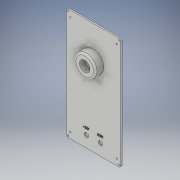
# Autodesk Inventor part: InnerDoorCover
Saved by Autodesk Inventor 2019 (Build 230136000, 136)
## iProperties
Created: 2019-02-25
Part Number: InnerDoorCover
Material: Generic
Document SubType Name: Modeling
Designer: garretthagen21
Density: 1 g/cm^3
Appearance: Default
Author: garretthagen21
Autodesk Inventor part; units mm, degrees
ref_plane "YZ Plane" through (0, 0, 0) normal (1, 0, 0) x (0, 1, 0)
ref_plane "XZ Plane" through (0, 0, 0) normal (0, 1, 0) x (-1, 0, 0)
ref_plane "XY Plane" through (0, 0, 0) normal (0, 0, 1) x (1, 0, 0)
sketch "Base" plane through (0, 0, 0) normal (0, 0, 1) x (1, 0, 0)
  line L0 (-5.5432, 7.38) -> (85.3888, 7.38)
  line L1 (88.5638, 4.205) -> (88.5638, -189.343)
  line L2 (85.3888, -192.518) -> (-5.5432, -192.518)
  line L3 (-8.7182, -189.343) -> (-8.7182, 4.205)
  arc A0 (-5.5432, 7.38) -> (-8.7182, 4.205) centre (-5.5432, 4.205) ccw
  arc A1 (88.5638, 4.205) -> (85.3888, 7.38) centre (85.3888, 4.205) ccw
  arc A2 (85.3888, -192.518) -> (88.5638, -189.343) centre (85.3888, -189.343) ccw
  arc A3 (-8.7182, -189.343) -> (-5.5432, -192.518) centre (-5.5432, -189.343) ccw
  point P0 (0, 0)
  point P1 (88.5638, -192.518)
  point P2 (88.5638, 7.38)
  point P3 (-8.7182, -192.518)
  dimension "d0" = 97.282
  dimension "d1" = 199.898
  dimension "d2" = 3.175
  constraints: 8 end point, 8 point on circle, 8 tangent, 6 point on line, 4 centre point, 3 equal radius, 2 parallel, 1 horizontal, 1 perpendicular
  measures "d0" distance of point (88.564, -192.518) point (-8.718, -192.518)
  measures "d1" distance of point (88.564, 7.38) point (88.564, -192.518)
  measures "d2" radius of A0
extrude "Extrusion1" add sketch "Base" along normal blind 2.54
sketch "Sketch2" plane through (0, 0, 2.54) normal (0, 0, 1) x (1, 0, 0)
  line L0 (85.3888, 7.38) -> (-5.5432, 7.38) projected
  line L1 (-8.7182, 4.205) -> (-8.7182, -189.343) projected
  line L2 (88.5638, -189.343) -> (88.5638, 4.205) projected
  line L3 (-5.5432, -192.518) -> (85.3888, -192.518) projected
  point P0 (0, 0)
  point P1 (-5.4162, 4.078)
  point P2 (85.2618, 4.078)
  point P3 (-5.4162, -189.216)
  point P4 (85.2618, -189.216)
  point P5 (-1.6062, -3.542)
  point P6 (81.4518, -3.542)
  point P7 (81.4518, -181.596)
  point P8 (-1.6062, -181.596)
  dimension "d5" = 3.302
  dimension "d6" = 3.302
  dimension "d7" = 3.302
  dimension "d8" = 3.302
  dimension "d9" = 3.302
  dimension "d10" = 3.302
  dimension "d11" = 3.302
  dimension "d12" = 3.302
  dimension "d13" = 10.922
  dimension "d14" = 7.112
  dimension "d15" = 7.112
  dimension "d16" = 10.922
  dimension "d17" = 10.922
  dimension "d18" = 7.112
  dimension "d19" = 10.922
  dimension "d20" = 7.112
  measures "d5" distance from line of L0 point (-5.416, 4.078)
  measures "d6" distance from line of L1 point (-5.416, 4.078)
  measures "d7" distance from line of point (85.262, 4.078) L0
  measures "d8" distance from line of point (85.262, 4.078) L2
  measures "d9" distance from line of L3 point (85.262, -189.216)
  measures "d10" distance from line of point (85.262, -189.216) L2
  measures "d11" distance from line of L1 point (-5.416, -189.216)
  measures "d12" distance from line of L3 point (-5.416, -189.216)
  measures "d13" distance from line of L0 point (-1.606, -3.542)
  measures "d14" distance from line of L1 point (-1.606, -3.542)
  measures "d15" distance from line of L2 point (81.452, -3.542)
  measures "d16" distance from line of L0 point (81.452, -3.542)
  measures "d17" distance from line of L3 point (81.452, -181.596)
  measures "d18" distance from line of L2 point (81.452, -181.596)
  measures "d19" distance from line of L3 point (-1.606, -181.596)
  measures "d20" distance from line of L1 point (-1.606, -181.596)
hole "ScrewHoles" at (-5.4162, 4.078, 2.54) at (85.2618, 4.078, 2.54) at (-5.4162, -189.216, 2.54) at (85.2618, -189.216, 2.54) at (81.4518, -181.596, 2.54) at (-1.6062, -181.596, 2.54) at (81.4518, -3.542, 2.54) at (-1.6062, -3.542, 2.54) direction (0, 0, -1) diameter 2.54 depth 2.54 tip angle 118
sketch "Sketch3" plane through (0, 0, 2.54) normal (0, 0, 1) x (1, 0, 0)
  line L0 (85.3888, -192.518) -> (-5.5432, -192.518) projected
  line L1 (39.9228, -192.518) -> (39.9228, -150.4359)
  line L2 (39.9228, -150.4359) -> (-8.7182, -150.4359)
  line L3 (-8.7182, -189.343) -> (-8.7182, 4.205) projected
  line L4 (39.9228, -150.4359) -> (88.5638, -150.4359)
  line L5 (88.5638, 4.205) -> (88.5638, -189.343) projected
  point P0 (0, 0)
  point P1 (27.2228, -171.9144)
  point P2 (52.6228, -171.9144)
  constraints: 6 end point, 3 point on line, 1 midpoint, 1 perpendicular, 1 vertical
hole "InputHoles" at (27.2228, -171.9144, 2.54) at (52.6228, -171.9144, 2.54) direction (0, 0, -1) diameter 7.747 depth 2.54 tip angle 118
sketch "Sketch4" plane through (0, 0, 2.54) normal (0, 0, 1) x (1, 0, 0)
  circle A0 centre (39.3518, -51.3692) radius 19.05
  point P0 (0, 0)
  dimension "d37" = 38.1
  constraints: 1 centre point
  measures "d37" diameter of A0
extrude "ButtonStand" add sketch "Sketch4" along normal blind 15.24
sketch "Sketch5" plane through (39.3518, -51.3692, 17.78) normal (0, 0, 1) x (1, 0, 0)
  circle A0 centre (0, 0) radius 19.05 projected
  point P0 (-39.3518, 51.3692)
  constraints: 1 coincident
hole "ButtonHole" at (39.3518, -51.3692, 17.78) direction (0, 0, -1) diameter 18.8976 end through all
fillet "Fillet1" radius 3.175 1 edges at (20.3018, -51.3692, 17.78)
sketch "Sketch6" plane through (0, 0, 2.54) normal (0, 0, 1) x (1, 0, 0)
  line L0 (22.0442, -158.7766) -> (32.2059, -158.7766) construction
  line L1 (32.2059, -158.7766) -> (32.2059, -161.8889) construction
  line L2 (32.2059, -161.8889) -> (22.0442, -161.8889) construction
  line L3 (22.0442, -161.8889) -> (22.0442, -158.7766) construction
  line L4 (47.3818, -158.6713) -> (57.415, -158.6713) construction
  line L5 (57.415, -158.6713) -> (57.415, -161.8477) construction
  line L6 (57.415, -161.8477) -> (47.3818, -161.8477) construction
  line L7 (47.3818, -161.8477) -> (47.3818, -158.6713) construction
  circle A0 centre (27.2228, -171.9144) radius 3.8735 projected
  circle A1 centre (52.6228, -171.9144) radius 3.8735 projected
  line L8 (24.7736, -160.7181) -> (23.7411, -160.7181)
  line L9 (23.7411, -160.7181) -> (23.7411, -161.7505)
  line L10 (23.7411, -161.7505) -> (23.4003, -161.7505)
  line L11 (23.4003, -161.7505) -> (23.4003, -160.7181)
  line L12 (23.4003, -160.7181) -> (22.3678, -160.7181)
  line L13 (22.3678, -160.7181) -> (22.3678, -160.3896)
  line L14 (22.3678, -160.3896) -> (23.4003, -160.3896)
  line L15 (23.4003, -160.3896) -> (23.4003, -159.3571)
  line L16 (23.4003, -159.3571) -> (23.7411, -159.3571)
  line L17 (23.7411, -159.3571) -> (23.7411, -160.3896)
  line L18 (23.7411, -160.3896) -> (24.7736, -160.3896)
  line L19 (24.7736, -160.3896) -> (24.7736, -160.7181)
  line L20 (27.0435, -161.8889) -> (25.5566, -161.8889)
  line L21 (25.5566, -161.8889) -> (25.5566, -161.5776)
  line L22 (25.5566, -161.5776) -> (26.1099, -161.5776)
  line L23 (26.1099, -161.5776) -> (26.1099, -159.5349)
  line L24 (26.1099, -159.5349) -> (25.5566, -159.5349)
  line L25 (25.5566, -159.5349) -> (25.5566, -159.2558)
  spline S0 degree 2 poles (25.5566, -159.2558) (25.8703, -159.2558) (26.1667, -159.078) (26.1864, -158.831) knots 0 0 0 1 2 2 2
  line L26 (26.1864, -158.831) -> (26.5026, -158.831)
  line L27 (26.5026, -158.831) -> (26.5026, -161.5776)
  line L28 (26.5026, -161.5776) -> (27.0435, -161.5776)
  line L29 (27.0435, -161.5776) -> (27.0435, -161.8889)
  line L30 (29.4839, -161.8889) -> (27.6042, -161.8889)
  line L31 (27.6042, -161.8889) -> (27.6042, -161.4566)
  spline S1 degree 2 poles (27.6042, -161.4566) (27.8068, -161.2664) (28.1674, -160.9132) (28.3403, -160.723) knots 0 0 0 1 2 2 2
  spline S2 degree 2 poles (28.3403, -160.723) (28.6886, -160.3402) (28.943, -159.8807) (28.943, -159.6362) knots 0 0 0 1 2 2 2
  spline S3 degree 2 poles (28.943, -159.6362) (28.943, -159.5078) (28.8639, -159.3151) (28.7923, -159.2534) knots 0 0 0 1 2 2 2
  spline S4 degree 2 poles (28.7923, -159.2534) (28.7207, -159.1916) (28.5329, -159.1299) (28.4193, -159.1299) knots 0 0 0 1 2 2 2
  spline S5 degree 2 poles (28.4193, -159.1299) (28.3106, -159.1299) (28.0883, -159.1842) (27.9871, -159.2262) knots 0 0 0 1 2 2 2
  spline S6 degree 2 poles (27.9871, -159.2262) (27.9006, -159.2608) (27.7401, -159.3596) (27.6907, -159.3941) knots 0 0 0 1 2 2 2
  line L32 (27.6907, -159.3941) -> (27.6684, -159.3941)
  line L33 (27.6684, -159.3941) -> (27.6684, -158.9594)
  spline S7 degree 2 poles (27.6684, -158.9594) (27.7944, -158.8977) (28.2464, -158.7766) (28.449, -158.7766) knots 0 0 0 1 2 2 2
  spline S8 degree 2 poles (28.449, -158.7766) (28.8763, -158.7766) (29.3579, -159.2287) (29.3579, -159.614) knots 0 0 0 1 2 2 2
  spline S9 degree 2 poles (29.3579, -159.614) (29.3579, -159.7943) (29.2739, -160.0956) (29.1998, -160.2241) knots 0 0 0 1 2 2 2
  spline S10 degree 2 poles (29.1998, -160.2241) (29.1257, -160.3575) (28.9109, -160.6193) (28.7923, -160.7452) knots 0 0 0 1 2 2 2
  spline S11 degree 2 poles (28.7923, -160.7452) (28.5996, -160.9552) (28.1279, -161.4047) (27.9871, -161.5357) knots 0 0 0 1 2 2 2
  line L34 (27.9871, -161.5357) -> (29.4839, -161.5357)
  line L35 (29.4839, -161.5357) -> (29.4839, -161.8889)
  line L36 (32.1886, -158.8409) -> (31.1388, -161.8889)
  line L37 (31.1388, -161.8889) -> (30.7016, -161.8889)
  line L38 (30.7016, -161.8889) -> (29.6519, -158.8409)
  line L39 (29.6519, -158.8409) -> (30.0866, -158.8409)
  line L40 (30.0866, -158.8409) -> (30.9313, -161.3726)
  line L41 (30.9313, -161.3726) -> (31.7761, -158.8409)
  line L42 (31.7761, -158.8409) -> (32.1886, -158.8409)
  line L43 (49.4566, -161.7835) -> (47.6905, -161.7835)
  line L44 (47.6905, -161.7835) -> (47.6905, -158.7355)
  line L45 (47.6905, -158.7355) -> (48.0956, -158.7355)
  line L46 (48.0956, -158.7355) -> (48.0956, -161.4229)
  line L47 (48.0956, -161.4229) -> (49.4566, -161.4229)
  line L48 (49.4566, -161.4229) -> (49.4566, -161.7835)
  spline S12 degree 2 poles (51.9315, -159.0838) (52.1044, -159.2863) (52.2971, -159.8791) (52.2971, -160.2595) knots 0 0 0 1 2 2 2
  spline S13 degree 2 poles (52.2971, -160.2595) (52.2971, -160.63) (52.1094, -161.2302) (51.9315, -161.4327) knots 0 0 0 1 2 2 2
  spline S14 degree 2 poles (51.9315, -161.4327) (51.7438, -161.6452) (51.2473, -161.8477) (50.9485, -161.8477) knots 0 0 0 1 2 2 2
  spline S15 degree 2 poles (50.9485, -161.8477) (50.6397, -161.8477) (50.1457, -161.6378) (49.9654, -161.4327) knots 0 0 0 1 2 2 2
  spline S16 degree 2 poles (49.9654, -161.4327) (49.79, -161.2302) (49.6023, -160.6349) (49.6023, -160.2595) knots 0 0 0 1 2 2 2
  spline S17 degree 2 poles (49.6023, -160.2595) (49.6023, -159.8766) (49.7925, -159.2937) (49.9679, -159.0838) knots 0 0 0 1 2 2 2
  spline S18 degree 2 poles (49.9679, -159.0838) (50.1457, -158.8812) (50.6422, -158.6713) (50.9485, -158.6713) knots 0 0 0 1 2 2 2
  spline S19 degree 2 poles (50.9485, -158.6713) (51.2597, -158.6713) (51.7586, -158.8886) (51.9315, -159.0838) knots 0 0 0 1 2 2 2
  spline S20 degree 2 poles (51.8747, -160.2595) (51.8747, -159.9581) (51.7438, -159.4913) (51.6253, -159.3382) knots 0 0 0 1 2 2 2
  spline S21 degree 2 poles (51.6253, -159.3382) (51.5042, -159.1801) (51.1634, -159.022) (50.9509, -159.022) knots 0 0 0 1 2 2 2
  spline S22 degree 2 poles (50.9509, -159.022) (50.7311, -159.022) (50.4001, -159.1752) (50.2742, -159.3382) knots 0 0 0 1 2 2 2
  spline S23 degree 2 poles (50.2742, -159.3382) (50.1531, -159.4938) (50.0247, -159.9631) (50.0247, -160.2595) knots 0 0 0 1 2 2 2
  spline S24 degree 2 poles (50.0247, -160.2595) (50.0247, -160.8597) (50.5286, -161.497) (50.9509, -161.497) knots 0 0 0 1 2 2 2
  spline S25 degree 2 poles (50.9509, -161.497) (51.3733, -161.497) (51.8747, -160.8597) (51.8747, -160.2595) knots 0 0 0 1 2 2 2
  spline S26 degree 2 poles (53.9323, -161.8378) (53.6359, -161.8378) (53.1344, -161.6378) (52.9517, -161.4377) knots 0 0 0 1 2 2 2
  spline S27 degree 2 poles (52.9517, -161.4377) (52.7689, -161.2401) (52.5688, -160.6473) (52.5688, -160.262) knots 0 0 0 1 2 2 2
  spline S28 degree 2 poles (52.5688, -160.262) (52.5688, -159.8791) (52.7639, -159.311) (52.9492, -159.1011) knots 0 0 0 1 2 2 2
  spline S29 degree 2 poles (52.9492, -159.1011) (53.132, -158.896) (53.6309, -158.6812) (53.9397, -158.6812) knots 0 0 0 1 2 2 2
  spline S30 degree 2 poles (53.9397, -158.6812) (54.0928, -158.6812) (54.362, -158.7256) (54.4757, -158.7602) knots 0 0 0 1 2 2 2
  spline S31 degree 2 poles (54.4757, -158.7602) (54.5745, -158.7923) (54.7795, -158.8837) (54.8807, -158.938) knots 0 0 0 1 2 2 2
  line L49 (54.8807, -158.938) -> (54.8807, -159.4271)
  line L50 (54.8807, -159.4271) -> (54.8486, -159.4271)
  spline S32 degree 2 poles (54.8486, -159.4271) (54.7943, -159.3777) (54.6263, -159.2394) (54.5053, -159.1727) knots 0 0 0 1 2 2 2
  spline S33 degree 2 poles (54.5053, -159.1727) (54.3892, -159.1085) (54.115, -159.027) (53.9372, -159.027) knots 0 0 0 1 2 2 2
  spline S34 degree 2 poles (53.9372, -159.027) (53.7421, -159.027) (53.3938, -159.1875) (53.2629, -159.3406) knots 0 0 0 1 2 2 2
  spline S35 degree 2 poles (53.2629, -159.3406) (53.1344, -159.4963) (52.9912, -159.968) (52.9912, -160.262) knots 0 0 0 1 2 2 2
  spline S36 degree 2 poles (52.9912, -160.262) (52.9912, -160.5757) (53.1418, -161.0277) (53.2728, -161.1833) knots 0 0 0 1 2 2 2
  spline S37 degree 2 poles (53.2728, -161.1833) (53.4012, -161.3339) (53.7445, -161.4871) (53.9372, -161.4871) knots 0 0 0 1 2 2 2
  spline S38 degree 2 poles (53.9372, -161.4871) (54.1126, -161.4871) (54.4114, -161.4006) (54.5275, -161.3364) knots 0 0 0 1 2 2 2
  spline S39 degree 2 poles (54.5275, -161.3364) (54.6387, -161.2722) (54.8042, -161.1388) (54.8511, -161.0919) knots 0 0 0 1 2 2 2
  line L51 (54.8511, -161.0919) -> (54.8807, -161.0919)
  line L52 (54.8807, -161.0919) -> (54.8807, -161.576)
  spline S40 degree 2 poles (54.8807, -161.576) (54.7795, -161.6229) (54.6016, -161.7094) (54.4757, -161.7489) knots 0 0 0 1 2 2 2
  spline S41 degree 2 poles (54.4757, -161.7489) (54.3423, -161.7934) (54.115, -161.8378) (53.9323, -161.8378) knots 0 0 0 1 2 2 2
  line L53 (57.4817, -161.7835) -> (56.9556, -161.7835)
  line L54 (56.9556, -161.7835) -> (55.8416, -160.3657)
  line L55 (55.8416, -160.3657) -> (55.6637, -160.5658)
  line L56 (55.6637, -160.5658) -> (55.6637, -161.7835)
  line L57 (55.6637, -161.7835) -> (55.2587, -161.7835)
  line L58 (55.2587, -161.7835) -> (55.2587, -158.7355)
  line L59 (55.2587, -158.7355) -> (55.6637, -158.7355)
  line L60 (55.6637, -158.7355) -> (55.6637, -160.136)
  line L61 (55.6637, -160.136) -> (56.9136, -158.7355)
  line L62 (56.9136, -158.7355) -> (57.4076, -158.7355)
  line L63 (57.4076, -158.7355) -> (56.1454, -160.0965)
  line L64 (56.1454, -160.0965) -> (57.4817, -161.7835)
  point P0 (0, 0)
  constraints: 4 other
emboss "Text" sketch "Sketch6" operation add depth 1.27 direction (0, 0, -1) contours L8 L9 L10 L11 L12 L13 L14 L15 L16 L17 L18 L19 | L20 L21 L22 L23 L24 L25 S0 L26 L27 L28 L29 | L30 L31 S1 S2 S3 S4 S5 S6 L32 L33 S7 S8 S9 S10 S11 L34 L35 | L36 L37 L38 L39 L40 L41 L42 | L43 L44 L45 L46 L47 L48 | S12 S13 S14 S15 S16 S17 S18 S19 | S26 S27 S28 S29 S30 S31 L49 L50 S32 S33 S34 S35 S36 S37 S38 S39 L51 L52 S40 S41 | L53 L54 L55 L56 L57 L58 L59 L60 L61 L62 L63 L64
sketch "Sketch7" plane through (0, 0, 0) normal (0, 0, -1) x (-1, 0, 0)
  circle A0 centre (-39.3518, -51.3692) radius 15.875 projected
  circle A1 centre (-39.3518, -51.3692) radius 13.97
  circle A2 centre (-39.3518, -51.3692) radius 9.4488
  point P0 (0, 0)
  dimension "d50" = 27.94
  constraints: 2 centre point, 2 coincident
  measures "d50" diameter of A1
extrude "ButtonSink" cut sketch "Sketch7" against normal blind 7.62 contours A1
body "Solid1"
